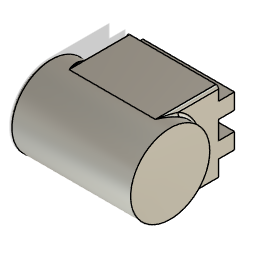
Link2 v28 (Autodesk Fusion 360 design; units mm, degrees)
Autodesk Fusion 360 part; units mm, degrees
sketch "Boceto1" plane through (0, 0, 0) normal (0, 0, 1) x (1, 0, 0)
  line L0 (0, 75) -> (-20, 75)
  line L1 (-20, 75) -> (-20, 50)
  line L2 (-20, 50) -> (-50, 50)
  line L3 (-50, 50) -> (-50, 20)
  line L4 (-50, 20) -> (-20, 20)
  line L5 (-20, 20) -> (-20, -15)
  line L6 (-20, -15) -> (-50, -15)
  line L7 (-50, -15) -> (-50, -45)
  line L8 (-50, -45) -> (-20, -45)
  line L9 (-20, -45) -> (-20, -75)
  line L10 (-20, -75) -> (95, -75)
  line L11 (95, -75) -> (95, 75)
  line L12 (95, 75) -> (0, 75)
  dimension "d22" = 25
  dimension "d24" = 30
  dimension "d25" = 35
  dimension "d26" = 30
  dimension "d27" = 30
  dimension "d28" = 30
  dimension "d33" = 115
  constraint horizontal L0
  constraint perpendicular L0 L1
  constraint perpendicular L1 L2
  constraint perpendicular L2 L3
  constraint perpendicular L3 L4
  constraint perpendicular L4 L5
  constraint perpendicular L5 L6
  constraint perpendicular L6 L7
  constraint perpendicular L7 L8
  constraint perpendicular L8 L9
  constraint perpendicular L9 L10
  constraint perpendicular L10 L11
  measures "d22" distance of L0.end L1.end
  measures "d24" distance of L2.end L3.end
  measures "d25" distance of L4.end L5.end
  measures "d26" distance of L5.end L6.end
  measures "d27" distance of L6.end L7.end
  measures "d28" distance of L8.end L9.end
  measures "d33" distance of L1 L11
sketch "Boceto6" plane through (0, 0, 0) normal (0, 0, 1) x (1, 0, 0)
extrude "Extruir6" add sketch "Boceto1" along normal blind 173.5
ref_plane "PlanoDeObra4" through (22.5, 0, 86.75) normal (0, 0, 1) x (1, 0, 0)
sketch "Boceto10" plane through (0, 0, 86.75) normal (0, 0, 1) x (1, 0, 0)
  circle A0 centre (95, 0) radius 75
  circle A1 centre (95, 0) radius 55
  dimension "d35" = 150
  dimension "d44" = 110
  constraint concentric A0 A1
  measures "d35" diameter of A0
  measures "d44" diameter of A1
extrude "Extruir8" add sketch "Boceto10" along normal blind 120 and the other way blind 110 contours A0 | A1
fillet "Empalme1" radius 5 1 edges at (25.0754, -27.1212, 206.75)
fillet "Fillet2" radius 5 4 edges at (37.5, 75, 0) (37.5, 75, 173.5) (20, 0, 173.5) (20, 0, 0)
extrude "Extrude9" cut sketch "Boceto10" along normal blind 100 and the other way blind 90 contours A1
move_body "Desplazar1" bodies 1 to x (0, 1, 0) y (0, 0, 1) z (1, 0, 0) at (-106.75, -95, 201.75)
move_body "Desplazar2" bodies 1 to x (1, 0, 0) y (0, -1, 0) z (0, 0, -1) at (0, -260, 373.5)
move_body "Desplazar3" bodies 1 to x (1, 0, 0) y (0, 1, 0) z (0, 0, 1) at (25, 0, -175)
move_body "Desplazar4" bodies 1 to x (1, 0, 0) y (0, 1, 0) z (0, 0, 1) at (0, 250, 0)
move_body "Desplazar5" bodies 1 to x (-1, 0, 0) y (0, -1, 0) z (0, 0, 1) at (-210, -20, 0)
move_body "Desplazar6" bodies 1 to x (0, -1, 0) y (1, 0, 0) z (0, 0, 1) at (-180, -240, 0)
move_body "Desplazar7" bodies 1 to x (1, 0, 0) y (0, 1, 0) z (0, 0, 1) at (115, -95, 0)
sketch "Sketch11" plane through (0, 0, 0) normal (0, 1, 0) x (1, 0, 0)
  line L0 (-190, 23.25) -> (-190, -11.75)
move_body "Move8" bodies 1 to x (1, 0, 0) y (0, 1, 0) z (0, 0, 1) at (190, 120, 5.75)
sketch "Sketch12" plane through (0, 0, 0) normal (0, 1, 0) x (1, 0, 0)
  line L0 (-30, 23.25) -> (-30, -11.75)
  dimension "d59" = 35
  dimension "d60" = 11.75
  dimension "d61" = 23.25
  constraint vertical L0
  measures "d59" distance of L0.start L0.end
  measures "d60" vertical distance of origin L0.end
  measures "d61" vertical distance of origin L0.start
sketch "Sketch13" plane through (0, 0, 0) normal (0, 0, 1) x (1, 0, 0)
  line L0 (-30, -33.25) -> (-30, 0)
  line L1 (-30, -33.25) -> (-30, -206.75)
  point P0 (-30, 0)
  dimension "d62" = 33.25
  dimension "d63" = 173.5
  constraint vertical L0
  constraint parallel L0 L1
  measures "d62" distance of L0.start P0
  measures "d63" distance of L0.start L1.end
sketch "Sketch14" plane through (0, 0, 77.5) normal (0, 0, 1) x (1, 0, 0)
  line L0 (0, -86.75) -> (87.1612, -86.75)
  spline S0 degree 3 poles (115, -91.75) (110.6901, -90.6372) (105.953, -89.4019) (96.4145, -87.4567) (91.6124, -86.75) (87.1612, -86.75) knots 0 0 0 0 1.335377 1.335377 2.670755 2.670755 2.670755 2.670755
  line L1 (115, -91.75) -> (115, 91.75)
  spline S1 degree 3 poles (87.1612, 86.75) (91.6124, 86.75) (96.4145, 87.4567) (105.953, 89.4019) (110.6901, 90.6372) (115, 91.75) knots 5.338444 5.338444 5.338444 5.338444 6.673822 6.673822 8.009199 8.009199 8.009199 8.009199
  line L2 (87.1612, 86.75) -> (0, 86.75)
  line L3 (0, 86.75) -> (0, -86.75)
move_body "Move9" bodies 1 to x (1, 0, 0) y (0, -1, 0) z (0, 0, -1) at (0, 0, 0)
sketch "Sketch15" plane through (0, 0, 72.5) normal (0, 0, 1) x (1, 0, 0)
  line L0 (0, -81.75) -> (115, -81.75)
  line L1 (115, -81.75) -> (115, 81.75)
  line L2 (115, 81.75) -> (0, 81.75)
  line L3 (0, 81.75) -> (0, -81.75)
  line L4 (130, 0) -> (130, 110)
  dimension "d64" = 110
  constraint parallel L1 L4
  measures "d64" distance of L4.start L4.end
sketch "Sketch16" plane through (0, 0, 72.5) normal (0, 0, 1) x (1, 0, 0)
  line L0 (0, -81.75) -> (115, -81.75)
  line L1 (115, -81.75) -> (115, 81.75)
  line L2 (115, 81.75) -> (0, 81.75)
  line L3 (0, 81.75) -> (0, -81.75)
  line L4 (115, 0) -> (190, 0)
  line L5 (115, 0) -> (-30, 0)
  line L6 (115, -91.75) -> (115, 91.75)
  line L7 (0, 86.75) -> (0, -86.75)
  dimension "d66" = 115
  constraint midpoint L1 L4.start
  constraint perpendicular L1 L4
  constraint perpendicular L3 L5
  measures "d66" distance of L6 L7
sketch "Sketch17" plane through (0, 0, 72.5) normal (0, 0, 1) x (1, 0, 0)
  line L0 (0, -81.75) -> (115, -81.75)
  line L1 (115, -81.75) -> (115, 81.75)
  line L2 (115, 81.75) -> (0, 81.75)
  line L3 (0, 81.75) -> (0, -81.75)
  line L4 (185, -120) -> (45, -120)
  point P0 (-30, 0)
  point P1 (130, 110)
  point P2 (0, 86.75)
  dimension "d67" = 110
  dimension "d68" = 120
  dimension "d69" = 86.75
  measures "d67" vertical distance of P0 P1
  measures "d68" distance of P0 L4
  measures "d69" vertical distance of P0 P2
